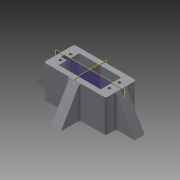
# Autodesk Inventor part: Servo Mount
Saved by Autodesk Inventor 2015 (Build 190159000, 159)
## iProperties
Created: 2016-12-13
Part Number: Servo Mount
Material: Generic
Document SubType Name: Modeling
Designer: Rudge-Top
Density: 1 g/cm^3
Appearance: Default
Author: Rudge-Top
Autodesk Inventor part; units mm, degrees
ref_plane "YZ Plane" through (0, 0, 0) normal (1, 0, 0) x (0, 1, 0)
ref_plane "XZ Plane" through (0, 0, 0) normal (0, 1, 0) x (-1, 0, 0)
ref_plane "XY Plane" through (0, 0, 0) normal (0, 0, 1) x (1, 0, 0)
sketch "Sketch1" plane through (0, 0, 0) normal (0, 1, 0) x (-1, 0, 0)
  line L0 (0, 0) -> (42, 0)
  line L1 (42, 0) -> (42, -20.5)
  line L2 (42, -20.5) -> (0, -20.5)
  line L3 (0, -20.5) -> (0, 0)
  line L4 (52, -25.5) -> (52, 5)
  line L5 (-10, 5) -> (-10, -25.5)
  line L6 (-10, 5) -> (52, 5)
  line L7 (52, -25.5) -> (-10, -25.5)
  dimension "d0" = 42
  dimension "d1" = 20.5
  dimension "d2" = 10
  dimension "d15" = 5
  dimension "d16" = 5
  constraints: 16 end point, 3 parallel, 3 perpendicular, 1 horizontal
  measures "d0" distance of L1.end L2.end
  measures "d1" distance of L0.end L1.end
  measures "d2" distance between parallel lines of L1 L4
  measures "d15" distance between parallel lines of L2 L7
  measures "d16" distance between parallel lines of L6 L0
extrude "Extrusion1" add sketch "Sketch1" along normal blind 29.5
sketch "Sketch2" plane through (0, 0, 0) normal (0, -1, 0) x (1, 0, 0)
  line L0 (-52, 5) -> (10, 5)
  line L1 (10, 5) -> (10, -25.5)
  line L2 (10, -25.5) -> (-52, -25.5)
  line L3 (-52, -25.5) -> (-52, 5)
  point P0 (0, 0)
  constraints: 8 end point, 2 parallel, 1 horizontal, 1 perpendicular
extrude "Extrusion2" add sketch "Sketch2" along normal blind 3
fillet "Fillet1" radius 2 4 edges at (-52, 13.25, -25.5) (10, 13.25, -25.5) (10, 13.25, 5) (-52, 13.25, 5)
sketch "Sketch3" plane through (0, 29.5, 0) normal (0, 1, 0) x (1, 0, 0)
  arc A0 (-52, -3) -> (-50, -5) centre (-50, -3) ccw projected
  arc A1 (8, -5) -> (10, -3) centre (8, -3) ccw projected
  line L0 (10, -3) -> (10, 23.5) projected
  arc A2 (10, 23.5) -> (8, 25.5) centre (8, 23.5) ccw projected
  arc A3 (-50, 25.5) -> (-52, 23.5) centre (-50, 23.5) ccw projected
  line L1 (-52, 23.5) -> (-52, -3) projected
  line L2 (-42, 0) -> (-42, 20.5) projected
  line L3 (-42, 20.5) -> (0, 20.5) projected
  line L4 (0, 20.5) -> (0, 0) projected
  line L5 (0, 0) -> (-42, 0) projected
  line L6 (-50, -5) -> (8, -5) projected
  line L7 (8, 25.5) -> (-50, 25.5) projected
  point P0 (3.5, 5.25)
  point P1 (3.5, 15.25)
  point P2 (-45.5, 5.25)
  point P3 (-45.5, 15.25)
  dimension "d8" = 10
  dimension "d10" = 3.5
  dimension "d11" = 10
  dimension "d12" = 3.5
  dimension "d17" = 10.25
  dimension "d18" = 10.25
  measures "d8" distance of point (-45.5, 5.25) point (-45.5, 15.25)
  measures "d10" distance from line of L2 point (-45.5, 15.25)
  measures "d11" distance of point (3.5, 15.25) point (3.5, 5.25)
  measures "d12" distance from line of L4 point (3.5, 5.25)
  measures "d17" distance from line of L6 point (3.5, 5.25)
  measures "d18" distance from line of L7 point (-45.5, 15.25)
hole "Hole1" at (3.5, 29.5, -5.25) at (3.5, 29.5, -15.25) at (-45.5, 29.5, -5.25) at (-45.5, 29.5, -15.25) direction (0, -1, 0) diameter 3 depth 10 tip angle 118
ref_plane "Work Plane1" through (-21, -3, 3) normal (1, 0, 0) x (0, 0, -1)
sketch "Sketch4" plane through (-21, -3, 3) normal (1, 0, 0) x (0, 0, -1)
  line L0 (0, 0) -> (0, 32.5) projected
  line L1 (26.5, 0) -> (0, 0) projected
  line L2 (26.5, 32.5) -> (26.5, 0) projected
  line L3 (0, 32.5) -> (26.5, 32.5) projected
  line L4 (28.5, 32.5) -> (26.5, 32.5) projected
  line L5 (26.5, 32.5) -> (26.5, 0) projected
  line L6 (26.5, 0) -> (28.5, 0) projected
  line L7 (28.5, 0) -> (28.5, 32.5) projected
  line L8 (28.5, 32.5) -> (47.2639, 0)
  line L9 (28.5, 32.5) -> (66.0278, 32.5) construction
  line L10 (47.2639, 0) -> (28.5, 0)
  point P0 (3, 3)
  dimension "d26" = 60
  constraints: 6 end point, 2 horizontal, 1 equal length
  measures "d26" angle of L8 L9
extrude "Extrusion3" add sketch "Sketch4" along normal mid plane 10 contours L7 L8 L10
ref_plane "Work Plane2" through (-50, -3, -10.25) normal (0, 0, -1) x (-1, 0, 0)
mirror "Mirror1" about plane through (-50, -3, -10.25) normal (0, 0, -1) of "Extrusion3"
sketch "Sketch5" plane through (-50, -3, -10.25) normal (0, 0, -1) x (-1, 0, 0)
  line L0 (-58, 32.5) -> (-60, 32.5) projected
  line L1 (-60, 32.5) -> (-60, 0) projected
  line L2 (-60, 0) -> (-58, 0) projected
  line L3 (-58, 0) -> (-58, 32.5) projected
  line L4 (-60, 32.5) -> (-78.7639, 0)
  line L5 (-60, 32.5) -> (-22.4722, 32.5) construction
  line L6 (-78.7639, 0) -> (-60, 0)
  line L7 (-60, 32.5) -> (-60, 0)
  point P0 (-50, 3)
  dimension "d29" = 240
  constraints: 8 end point, 2 horizontal, 1 collinear, 1 equal length
extrude "Extrusion4" add sketch "Sketch5" along normal mid plane 10 contours L1 L6 L4
mirror "Mirror2" about plane through (-21, -3, 3) normal (1, 0, 0) of "Extrusion4"
fillet "Fillet2" radius 2 8 edges at (10, 13.25, -15.25) (10, 13.25, -5.25) (-16, 13.25, -25.5) (-26, 13.25, -25.5) (-52, 13.25, -15.25) (-52, 13.25, -5.25) (-26, 13.25, 5) (-16, 13.25, 5)
sketch "Sketch6" plane through (0, -3, 0) normal (0, -1, 0) x (1, 0, 0)
  line L0 (-42, -20.5) -> (0, -20.5)
  line L1 (0, -20.5) -> (0, 0)
  line L2 (0, 0) -> (-42, 0)
  line L3 (-42, 0) -> (-42, -20.5)
  line L4 (-50, -25.5) -> (-28, -25.5) projected
  line L5 (-52, 3) -> (-52, -3.25) projected
  point P0 (0, 0)
  dimension "d33" = 42
  dimension "d34" = 20.5
  dimension "d35" = 5
  dimension "d36" = 10
  constraints: 8 end point, 2 parallel, 1 horizontal, 1 perpendicular
  measures "d33" distance of L2.end L1.end
  measures "d34" distance of L1.end L0.end
  measures "d35" distance between parallel lines of L4 L0
  measures "d36" distance between parallel lines of L5 L3
extrude "Extrusion5" cut sketch "Sketch6" against normal blind 3
sketch "Sketch7" plane through (0, 29.5, 0) normal (0, 1, 0) x (1, 0, 0)
  circle A0 centre (-45.5, 5.25) radius 1.5 projected
  circle A1 centre (3.5, 5.25) radius 1.5 projected
  circle A2 centre (3.5, 15.25) radius 1.5 projected
  circle A3 centre (-45.5, 15.25) radius 1.5 projected
  arc A4 (-52, -3) -> (-50, -5) centre (-50, -3) ccw projected
  line L0 (-50, -5) -> (-28, -5) projected
  line L1 (-28, -5) -> (-14, -5) projected
  line L2 (-14, -5) -> (8, -5) projected
  arc A5 (8, -5) -> (10, -3) centre (8, -3) ccw projected
  line L3 (10, -3) -> (10, 3.25) projected
  line L4 (10, 3.25) -> (10, 17.25) projected
  line L5 (10, 17.25) -> (10, 23.5) projected
  arc A6 (10, 23.5) -> (8, 25.5) centre (8, 23.5) ccw projected
  line L6 (8, 25.5) -> (-14, 25.5) projected
  line L7 (-14, 25.5) -> (-28, 25.5) projected
  line L8 (-28, 25.5) -> (-50, 25.5) projected
  arc A7 (-50, 25.5) -> (-52, 23.5) centre (-50, 23.5) ccw projected
  line L9 (-52, 23.5) -> (-52, 17.25) projected
  line L10 (-52, 17.25) -> (-52, 3.25) projected
  line L11 (-52, 3.25) -> (-52, -3) projected
  line L12 (-42, 0) -> (-42, 20.5) projected
  line L13 (-42, 20.5) -> (0, 20.5) projected
  line L14 (0, 20.5) -> (0, 0) projected
  line L15 (0, 0) -> (-42, 0) projected
  line L16 (-42, 12.1833) -> (-48, 12.1833)
  line L17 (-48, 12.1833) -> (-48, 8.1833)
  line L18 (-48, 8.1833) -> (-42, 8.1833)
  line L19 (-42, 8.1833) -> (-42, 12.1833)
  line L20 (-42, 10.1833) -> (-45.1833, 10.1833)
  line L21 (-42, 10.1833) -> (-38.8167, 10.1833) construction
  dimension "d39" = 6
  dimension "d40" = 4
  dimension "d41" = 180
  constraints: 12 end point, 2 horizontal, 2 parallel, 1 collinear, 1 midpoint, 1 perpendicular, 1 point on line
  measures "d39" distance of L18.end L17.end
  measures "d40" distance of L17.end L16.end
  measures "d41" angle of L20 L21
extrude "Extrusion6" cut sketch "Sketch7" against normal blind 40 contours L18 L17 L16 L12
fillet "Fillet3" radius 0.5 2 edges at (-42, 13.25, -12.1833) (-42, 13.25, -8.1833)
ref_plane "Work Plane3" through (-21, -3, 3) normal (1, 0, 0) x (0, 0, -1)
body "Solid1"
